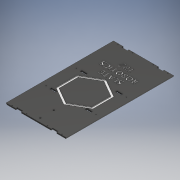
# Autodesk Inventor part: BA11
Saved by Autodesk Inventor 2017 (Build 210142000, 142)
## iProperties
Created: 2019-05-29
Part Number: BA11
Material: Wood (Cherry)
Document SubType Name: Modeling
Designer: Dell
Density: 0.63 g/cm^3
Appearance: Smooth - Black
Mass: 641.872 g
Surface Area: 3346.2 cm^2
Volume: 1018.84 cm^3
Author: Dell
Autodesk Inventor part; units mm, degrees
ref_plane "YZ Plane" through (0, 0, 0) normal (1, 0, 0) x (0, 1, 0)
ref_plane "XZ Plane" through (0, 0, 0) normal (0, 1, 0) x (-1, 0, 0)
ref_plane "XY Plane" through (0, 0, 0) normal (0, 0, 1) x (1, 0, 0)
sketch "Sketch1" plane through (0, 0, 0) normal (0, 0, 1) x (1, 0, 0)
  line L0 (0, 0) -> (303.5592, 0)
  line L1 (303.5592, 0) -> (303.5592, 539.75)
  line L2 (303.5592, 539.75) -> (0, 539.75)
  line L3 (0, 539.75) -> (0, 0)
  dimension "d0" = 539.75
  dimension "d1" = 303.5592
  constraints: 8 end point, 2 parallel, 1 horizontal, 1 perpendicular
  measures "d0" distance of L1.end L0.end
  measures "d1" distance of L1.end L2.end
extrude "Extrusion1" add sketch "Sketch1" along normal blind 6.35
sketch "Sketch2" plane through (0, 539.75, 0) normal (0, 1, 0) x (1, 0, 0)
  line L0 (0, -6.35) -> (303.5592, -6.35) projected
  line L1 (0, -6.35) -> (3.6662, 0)
  line L2 (0, 0) -> (303.5592, 0) projected
  line L3 (0, 0) -> (3.6662, 0)
  line L4 (0, 0) -> (0, -6.35)
  line L5 (303.5592, -6.35) -> (299.8931, 0)
  line L6 (303.5592, 0) -> (299.8931, 0)
  line L7 (303.5592, 0) -> (303.5592, -6.35) projected
  line L8 (303.5592, 0) -> (303.5592, -6.35)
  dimension "d4" = 30
  dimension "d5" = 30
  constraints: 12 end point, 2 collinear, 2 point on line, 1 perpendicular, 1 vertical
  measures "d4" angle of L4 L1
  measures "d5" angle of L5 L7
extrude "Extrusion2" cut sketch "Sketch2" against normal through all contours L4 L2 L1 | L5 L2 L7
sketch "Sketch3" plane through (0, 0, 6.35) normal (0, 0, 1) x (1, 0, 0)
  line L0 (50.1796, 532.13) -> (75.5796, 532.13)
  line L1 (75.5796, 532.13) -> (75.5796, 539.75)
  line L2 (75.5796, 539.75) -> (50.1796, 539.75)
  line L3 (50.1796, 539.75) -> (50.1796, 532.13)
  line L4 (303.5592, 539.75) -> (0, 539.75) projected
  line L5 (227.9796, 539.75) -> (253.3796, 539.75)
  line L6 (253.3796, 539.75) -> (253.3796, 532.13)
  line L7 (253.3796, 532.13) -> (227.9796, 532.13)
  line L8 (227.9796, 532.13) -> (227.9796, 539.75)
  line L9 (75.5796, 532.13) -> (227.9796, 532.13) construction
  line L10 (0, 0) -> (303.5592, 0) projected
  line L11 (50.1796, 0) -> (75.5796, 0)
  line L12 (75.5796, 0) -> (75.5796, 7.62)
  line L13 (75.5796, 7.62) -> (50.1796, 7.62)
  line L14 (50.1796, 7.62) -> (50.1796, 0)
  line L15 (253.3796, 0) -> (227.9796, 0)
  line L16 (227.9796, 0) -> (227.9796, 7.62)
  line L17 (227.9796, 7.62) -> (253.3796, 7.62)
  line L18 (253.3796, 7.62) -> (253.3796, 0)
  point P0 (151.7796, 532.13)
  point P1 (151.7796, 539.75)
  dimension "d8" = 7.62
  dimension "d9" = 25.4
  dimension "d10" = 25.4
  dimension "d11" = 152.4
  dimension "d14" = 7.62
  constraints: 34 end point, 8 parallel, 5 point on line, 5 vertical alignment, 4 horizontal, 4 perpendicular, 2 midpoint, 1 collinear, 1 horizontal alignment
  measures "d8" distance of L2.end L0.start
  measures "d9" distance of L0.start L0.end
  measures "d10" distance of L6.end L7.end
  measures "d11" distance of L0.end L7.end
  measures "d14" distance of L13.end L11.start
extrude "Extrusion3" cut sketch "Sketch3" against normal through all
sketch "Sketch4" plane through (0, 0, 6.35) normal (0, 0, 1) x (1, 0, 0)
  line L0 (50.1796, 330.2) -> (75.5796, 330.2)
  line L1 (75.5796, 330.2) -> (75.5796, 323.85)
  line L2 (75.5796, 323.85) -> (50.1796, 323.85)
  line L3 (50.1796, 323.85) -> (50.1796, 330.2)
  line L4 (227.9796, 330.2) -> (253.3796, 330.2)
  line L5 (253.3796, 330.2) -> (253.3796, 323.85)
  line L6 (253.3796, 323.85) -> (227.9796, 323.85)
  line L7 (227.9796, 323.85) -> (227.9796, 330.2)
  line L8 (75.5796, 532.13) -> (50.1796, 532.13) projected
  line L9 (253.3796, 532.13) -> (227.9796, 532.13) projected
  line L10 (227.9796, 539.75) -> (75.5796, 539.75) projected
  point P0 (0, 0)
  point P1 (62.8796, 330.2)
  point P2 (62.8796, 532.13)
  point P3 (240.6796, 330.2)
  point P4 (240.6796, 532.13)
  dimension "d15" = 25.4
  dimension "d16" = 6.35
  dimension "d17" = 25.4
  dimension "d18" = 6.35
  dimension "d19" = 209.55
  constraints: 16 end point, 4 midpoint, 4 parallel, 2 horizontal, 2 perpendicular, 2 vertical alignment, 1 horizontal alignment
  measures "d15" distance of L1.end L2.end
  measures "d16" distance of L0.end L1.end
  measures "d17" distance of L5.end L6.end
  measures "d18" distance of L4.end L5.end
  measures "d19" distance between parallel lines of L10 L0
extrude "Extrusion4" cut sketch "Sketch4" against normal through all
sketch "Sketch5" plane through (0, 0, 6.35) normal (0, 0, 1) x (1, 0, 0)
  line L0 (50.1796, 177.8) -> (75.5796, 177.8)
  line L1 (75.5796, 177.8) -> (75.5796, 171.45)
  line L2 (75.5796, 171.45) -> (50.1796, 171.45)
  line L3 (50.1796, 171.45) -> (50.1796, 177.8)
  line L4 (227.9796, 177.8) -> (253.3796, 177.8)
  line L5 (253.3796, 177.8) -> (253.3796, 171.45)
  line L6 (253.3796, 171.45) -> (227.9796, 171.45)
  line L7 (227.9796, 171.45) -> (227.9796, 177.8)
  line L8 (50.1796, 7.62) -> (75.5796, 7.62) projected
  line L9 (227.9796, 7.62) -> (253.3796, 7.62) projected
  line L10 (0, 0) -> (50.1796, 0) projected
  point P0 (62.8796, 171.45)
  point P1 (62.8796, 7.62)
  point P2 (240.6796, 7.62)
  point P3 (240.6796, 171.45)
  dimension "d22" = 25.4
  dimension "d23" = 6.35
  dimension "d24" = 25.4
  dimension "d25" = 6.35
  dimension "d27" = 177.8
  constraints: 16 end point, 4 midpoint, 4 parallel, 2 horizontal, 2 perpendicular, 2 vertical alignment, 1 horizontal alignment
  measures "d22" distance of L1.end L2.end
  measures "d23" distance of L0.end L1.end
  measures "d24" distance of L5.end L6.end
  measures "d25" distance of L4.end L5.end
  measures "d27" distance between parallel lines of L10 L0
extrude "Extrusion5" cut sketch "Sketch5" against normal through all
sketch "Sketch6" plane through (0, 0, 6.35) normal (0, 0, 1) x (1, 0, 0)
  line L0 (301.7796, 359.75) -> (1.7796, 359.75) construction
  line L1 (1.7796, 359.75) -> (1.7796, 469.75) construction
  line L2 (301.7796, 469.75) -> (301.7796, 359.75) construction
  line L3 (1.7796, 469.75) -> (301.7796, 469.75) construction
  line L4 (151.7796, 359.75) -> (151.7796, 414.75) construction
  line L5 (151.7796, 414.75) -> (1.7796, 414.75) construction
  line L6 (227.9796, 539.75) -> (75.5796, 539.75) projected
  line L7 (151.7796, 138.1902) -> (59.2796, 191.5951)
  line L8 (59.2796, 191.5951) -> (59.2796, 298.4049)
  line L9 (59.2796, 298.4049) -> (151.7796, 351.8098)
  line L10 (151.7796, 351.8098) -> (244.2796, 298.4049)
  line L11 (244.2796, 298.4049) -> (244.2796, 191.5951)
  line L12 (244.2796, 191.5951) -> (151.7796, 138.1902)
  line L13 (151.7796, 149.9681) -> (69.4796, 197.4841)
  line L14 (69.4796, 197.4841) -> (69.4796, 292.5159)
  line L15 (69.4796, 292.5159) -> (151.7796, 340.0319)
  line L16 (151.7796, 340.0319) -> (234.0796, 292.5159)
  line L17 (234.0796, 292.5159) -> (234.0796, 197.4841)
  line L18 (234.0796, 197.4841) -> (151.7796, 149.9681)
  line L19 (75.5796, 0) -> (227.9796, 0) projected
  line L20 (205.0313, 387.3542) -> (205.0313, 383.0696)
  spline S0 degree 2 poles (205.0313, 383.0696) (202.1048, 384.2937) (199.2165, 384.7719) (198.0114, 384.7719) knots 0 0 0 1 2 2 2
  spline S1 degree 2 poles (198.0114, 384.7719) (195.8309, 384.7719) (193.6694, 382.8209) (193.6694, 381.4437) knots 0 0 0 1 2 2 2
  spline S2 degree 2 poles (193.6694, 381.4437) (193.6694, 380.3917) (194.2624, 379.55) knots 0 0 0 1 1 1
  spline S3 degree 2 poles (194.2624, 379.55) (194.8745, 378.7276) (197.2272, 377.4077) knots 0 0 0 1 1 1
  line L21 (197.2272, 377.4077) -> (198.9104, 376.4705)
  spline S4 degree 2 poles (198.9104, 376.4705) (202.5256, 374.4621) (203.788, 372.7597) knots 0 0 0 1 1 1
  spline S5 degree 2 poles (203.788, 372.7597) (205.0887, 371.0573) (205.0887, 368.8194) knots 0 0 0 1 1 1
  spline S6 degree 2 poles (205.0887, 368.8194) (205.0887, 365.9885) (200.7658, 361.9716) (196.7299, 361.9716) knots 0 0 0 1 2 2 2
  spline S7 degree 2 poles (196.7299, 361.9716) (193.7077, 361.9716) (189.9204, 362.8324) knots 0 0 0 1 1 1
  line L22 (189.9204, 362.8324) -> (189.9204, 366.8301)
  spline S8 degree 2 poles (189.9204, 366.8301) (193.8033, 365.3955) (196.0795, 365.3955) knots 0 0 0 1 1 1
  spline S9 degree 2 poles (196.0795, 365.3955) (197.9732, 365.3955) (199.9433, 367.0405) (199.9433, 368.1882) knots 0 0 0 1 2 2 2
  spline S10 degree 2 poles (199.9433, 368.1882) (199.9433, 369.068) (199.3313, 369.814) knots 0 0 0 1 1 1
  spline S11 degree 2 poles (199.3313, 369.814) (198.7574, 370.5791) (196.4047, 371.8989) knots 0 0 0 1 1 1
  line L23 (196.4047, 371.8989) -> (194.6067, 372.8936)
  spline S12 degree 2 poles (194.6067, 372.8936) (190.456, 375.208) (189.3274, 376.9104) knots 0 0 0 1 1 1
  spline S13 degree 2 poles (189.3274, 376.9104) (188.1989, 378.6319) (188.1989, 380.7742) knots 0 0 0 1 1 1
  spline S14 degree 2 poles (188.1989, 380.7742) (188.1989, 383.8538) (192.8852, 388.1958) (197.9923, 388.1958) knots 0 0 0 1 2 2 2
  spline S15 degree 2 poles (197.9923, 388.1958) (201.0145, 388.1958) (205.0313, 387.3542) knots 0 0 0 1 1 1
  line L24 (183.876, 387.5837) -> (183.876, 362.5837)
  line L25 (183.876, 362.5837) -> (178.6733, 362.5837)
  line L26 (178.6733, 362.5837) -> (178.6733, 384.0451)
  line L27 (178.6733, 384.0451) -> (167.5218, 384.0451)
  line L28 (167.5218, 384.0451) -> (167.5218, 387.5837)
  line L29 (167.5218, 387.5837) -> (183.876, 387.5837)
  line L30 (166.508, 387.5837) -> (156.8102, 362.5837)
  line L31 (156.8102, 362.5837) -> (151.5883, 362.5837)
  line L32 (151.5883, 362.5837) -> (141.8523, 387.5837)
  line L33 (141.8523, 387.5837) -> (147.1889, 387.5837)
  line L34 (147.1889, 387.5837) -> (149.7903, 380.9081)
  line L35 (149.7903, 380.9081) -> (160.1193, 380.9081)
  line L36 (160.1193, 380.9081) -> (162.7207, 387.5837)
  line L37 (162.7207, 387.5837) -> (166.508, 387.5837)
  line L38 (158.8378, 377.5799) -> (151.091, 377.5799)
  line L39 (151.091, 377.5799) -> (154.9548, 367.6143)
  line L40 (154.9548, 367.6143) -> (158.8378, 377.5799)
  line L41 (132.0971, 387.5837) -> (132.0971, 366.0267)
  line L42 (132.0971, 366.0267) -> (141.0489, 366.0267)
  line L43 (141.0489, 366.0267) -> (141.0489, 362.5837)
  line L44 (141.0489, 362.5837) -> (117.9426, 362.5837)
  line L45 (117.9426, 362.5837) -> (117.9426, 366.0267)
  line L46 (117.9426, 366.0267) -> (126.8944, 366.0267)
  line L47 (126.8944, 366.0267) -> (126.8944, 387.5837)
  line L48 (126.8944, 387.5837) -> (132.0971, 387.5837)
  line L49 (114.4613, 387.5837) -> (114.4613, 362.5837)
  line L50 (114.4613, 362.5837) -> (98.4514, 362.5837)
  line L51 (98.4514, 362.5837) -> (98.4514, 366.0267)
  line L52 (98.4514, 366.0267) -> (109.2586, 366.0267)
  line L53 (109.2586, 366.0267) -> (109.2586, 372.9892)
  line L54 (109.2586, 372.9892) -> (100.3259, 372.9892)
  line L55 (100.3259, 372.9892) -> (100.3259, 376.4322)
  line L56 (100.3259, 376.4322) -> (109.2586, 376.4322)
  line L57 (109.2586, 376.4322) -> (109.2586, 384.0451)
  line L58 (109.2586, 384.0451) -> (97.648, 384.0451)
  line L59 (97.648, 384.0451) -> (97.648, 387.5837)
  line L60 (97.648, 387.5837) -> (114.4613, 387.5837)
  line L61 (239.7961, 427.5402) -> (239.7961, 402.5402)
  line L62 (239.7961, 402.5402) -> (230.4426, 402.5402)
  spline S16 degree 2 poles (230.4426, 402.5402) (227.5734, 402.5402) (224.5703, 403.9748) (222.8297, 406.9014) (222.8297, 408.7376) knots 0 0 0 1 2 3 3 3
  spline S17 degree 2 poles (222.8297, 408.7376) (222.8297, 410.9373) (225.3546, 414.8394) (227.669, 415.8723) knots 0 0 0 1 2 2 2
  line L63 (227.669, 415.8723) -> (219.5015, 427.5402)
  line L64 (219.5015, 427.5402) -> (225.8328, 427.5402)
  line L65 (225.8328, 427.5402) -> (232.0493, 417.326)
  line L66 (232.0493, 417.326) -> (234.8993, 417.326)
  line L67 (234.8993, 417.326) -> (234.8993, 427.5402)
  line L68 (234.8993, 427.5402) -> (239.7961, 427.5402)
  line L69 (234.8993, 413.9021) -> (233.7134, 413.9021)
  spline S18 degree 2 poles (233.7134, 413.9021) (230.5, 413.9021) (228.0325, 411.0903) (228.0325, 409.3115) knots 0 0 0 1 2 2 2
  spline S19 degree 2 poles (228.0325, 409.3115) (228.0325, 407.7812) (230.0218, 405.9641) (233.0822, 405.9641) knots 0 0 0 1 2 2 2
  line L70 (233.0822, 405.9641) -> (234.8993, 405.9641)
  line L71 (234.8993, 405.9641) -> (234.8993, 413.9021)
  spline S20 degree 2 poles (204.8114, 428.1523) (208.7134, 428.1523) (214.49, 424.9197) (217.4931, 418.8753) (217.4931, 415.0307) knots 0 0 0 1 2 3 3 3
  spline S21 degree 2 poles (217.4931, 415.0307) (217.4931, 411.2242) (214.49, 405.1416) (208.6752, 401.9281) (204.8114, 401.9281) knots 0 0 0 1 2 3 3 3
  spline S22 degree 2 poles (204.8114, 401.9281) (200.9667, 401.9281) (195.1518, 405.1416) (192.1488, 411.2242) (192.1488, 415.0307) knots 0 0 0 1 2 3 3 3
  spline S23 degree 2 poles (192.1488, 415.0307) (192.1488, 418.8753) (195.1518, 424.9197) (200.9093, 428.1523) (204.8114, 428.1523) knots 0 0 0 1 2 3 3 3
  spline S24 degree 2 poles (204.8114, 424.7284) (201.1962, 424.7284) (197.6767, 418.8371) (197.6767, 415.0307) knots 0 0 0 1 2 2 2
  spline S25 degree 2 poles (197.6767, 415.0307) (197.6767, 411.2051) (201.2153, 405.352) (204.8114, 405.352) knots 0 0 0 1 2 2 2
  spline S26 degree 2 poles (204.8114, 405.352) (208.4265, 405.352) (211.9651, 411.2051) (211.9651, 415.0307) knots 0 0 0 1 2 2 2
  spline S27 degree 2 poles (211.9651, 415.0307) (211.9651, 418.8371) (208.4456, 424.7284) (204.8114, 424.7284) knots 0 0 0 1 2 2 2
  line L72 (187.4816, 427.5402) -> (187.4816, 402.5402)
  line L73 (187.4816, 402.5402) -> (179.0462, 402.5402)
  spline S28 degree 2 poles (179.0462, 402.5402) (175.9858, 402.5402) (173.0593, 403.9174) (171.3951, 406.5953) (171.3951, 408.1064) knots 0 0 0 1 2 3 3 3
  spline S29 degree 2 poles (171.3951, 408.1064) (171.3951, 409.9809) (173.9965, 413.4239) (177.363, 414.476) knots 0 0 0 1 2 2 2
  spline S30 degree 2 poles (177.363, 414.476) (174.6851, 415.1454) (171.8542, 417.0965) (170.3814, 419.8126) (170.3814, 421.362) knots 0 0 0 1 2 3 3 3
  spline S31 degree 2 poles (170.3814, 421.362) (170.3814, 423.0452) (172.1029, 425.9717) (175.1251, 427.5402) (178.262, 427.5402) knots 0 0 0 1 2 3 3 3
  line L74 (178.262, 427.5402) -> (187.4816, 427.5402)
  line L75 (182.4892, 424.0016) -> (181.4946, 424.0016)
  spline S32 degree 2 poles (181.4946, 424.0016) (178.7785, 424.0016) (176.8083, 423.2939) (175.8137, 421.7063) (175.8137, 420.7307) knots 0 0 0 1 2 3 3 3
  spline S33 degree 2 poles (175.8137, 420.7307) (175.8137, 418.8753) (179.0845, 416.2931) (181.5902, 416.2931) knots 0 0 0 1 2 2 2
  line L76 (181.5902, 416.2931) -> (182.4892, 416.2931)
  line L77 (182.4892, 416.2931) -> (182.4892, 424.0016)
  line L78 (182.4892, 412.9457) -> (181.3798, 412.9457)
  spline S34 degree 2 poles (181.3798, 412.9457) (179.008, 412.9457) (176.6744, 410.593) (176.6744, 408.9098) knots 0 0 0 1 2 2 2
  spline S35 degree 2 poles (176.6744, 408.9098) (176.6744, 408.0108) (177.363, 406.6909) (179.1036, 405.9641) (181.552, 405.9641) knots 0 0 0 1 2 3 3 3
  line L79 (181.552, 405.9641) -> (182.4892, 405.9641)
  line L80 (182.4892, 405.9641) -> (182.4892, 412.9457)
  spline S36 degree 2 poles (154.5627, 428.1523) (158.4648, 428.1523) (164.2414, 424.9197) (167.2444, 418.8753) (167.2444, 415.0307) knots 0 0 0 1 2 3 3 3
  spline S37 degree 2 poles (167.2444, 415.0307) (167.2444, 411.2242) (164.2414, 405.1416) (158.4265, 401.9281) (154.5627, 401.9281) knots 0 0 0 1 2 3 3 3
  spline S38 degree 2 poles (154.5627, 401.9281) (150.718, 401.9281) (144.9032, 405.1416) (141.9001, 411.2242) (141.9001, 415.0307) knots 0 0 0 1 2 3 3 3
  spline S39 degree 2 poles (141.9001, 415.0307) (141.9001, 418.8753) (144.9032, 424.9197) (150.6606, 428.1523) (154.5627, 428.1523) knots 0 0 0 1 2 3 3 3
  spline S40 degree 2 poles (154.5627, 424.7284) (150.9475, 424.7284) (147.428, 418.8371) (147.428, 415.0307) knots 0 0 0 1 2 2 2
  spline S41 degree 2 poles (147.428, 415.0307) (147.428, 411.2051) (150.9667, 405.352) (154.5627, 405.352) knots 0 0 0 1 2 2 2
  spline S42 degree 2 poles (154.5627, 405.352) (158.1778, 405.352) (161.7165, 411.2051) (161.7165, 415.0307) knots 0 0 0 1 2 2 2
  spline S43 degree 2 poles (161.7165, 415.0307) (161.7165, 418.8371) (158.197, 424.7284) (154.5627, 424.7284) knots 0 0 0 1 2 2 2
  line L81 (131.0164, 427.5402) -> (131.0164, 405.9832)
  line L82 (131.0164, 405.9832) -> (139.9682, 405.9832)
  line L83 (139.9682, 405.9832) -> (139.9682, 402.5402)
  line L84 (139.9682, 402.5402) -> (116.8619, 402.5402)
  line L85 (116.8619, 402.5402) -> (116.8619, 405.9832)
  line L86 (116.8619, 405.9832) -> (125.8137, 405.9832)
  line L87 (125.8137, 405.9832) -> (125.8137, 427.5402)
  line L88 (125.8137, 427.5402) -> (131.0164, 427.5402)
  line L89 (113.3806, 427.5402) -> (113.3806, 402.5402)
  line L90 (113.3806, 402.5402) -> (108.1778, 402.5402)
  line L91 (108.1778, 402.5402) -> (108.1778, 427.5402)
  line L92 (108.1778, 427.5402) -> (113.3806, 427.5402)
  spline S44 degree 2 poles (81.8006, 426.5456) (83.4456, 427.2724) (85.8749, 427.808) (88.9544, 428.1523) (90.4655, 428.1523) knots 0 0 0 1 2 3 3 3
  spline S45 degree 2 poles (90.4655, 428.1523) (97.0264, 428.1523) (103.4724, 420.769) (103.4724, 415.0307) knots 0 0 0 1 2 2 2
  spline S46 degree 2 poles (103.4724, 415.0307) (103.4724, 409.2923) (97.0455, 401.9281) (90.1404, 401.9281) knots 0 0 0 1 2 2 2
  spline S47 degree 2 poles (90.1404, 401.9281) (86.0661, 401.9281) (82.0302, 402.8845) knots 0 0 0 1 1 1
  line L93 (82.0302, 402.8845) -> (82.0302, 406.9587)
  spline S48 degree 2 poles (82.0302, 406.9587) (83.9812, 406.2893) (86.4487, 405.658) (88.6484, 405.352) (89.7578, 405.352) knots 0 0 0 1 2 3 3 3
  spline S49 degree 2 poles (89.7578, 405.352) (94.0616, 405.352) (97.9445, 410.8799) (97.9445, 414.9733) knots 0 0 0 1 2 2 2
  spline S50 degree 2 poles (97.9445, 414.9733) (97.9445, 419.2579) (93.5451, 424.5563) (89.184, 424.5563) knots 0 0 0 1 2 2 2
  spline S51 degree 2 poles (89.184, 424.5563) (85.5497, 424.5563) (81.8006, 422.72) knots 0 0 0 1 1 1
  line L94 (81.8006, 422.72) -> (81.8006, 426.5456)
  line L95 (78.6828, 427.3107) -> (78.6828, 423.0261)
  spline S52 degree 2 poles (78.6828, 423.0261) (75.7563, 424.2502) (72.868, 424.7284) (71.6629, 424.7284) knots 0 0 0 1 2 2 2
  spline S53 degree 2 poles (71.6629, 424.7284) (69.4824, 424.7284) (67.3209, 422.7774) (67.3209, 421.4002) knots 0 0 0 1 2 2 2
  spline S54 degree 2 poles (67.3209, 421.4002) (67.3209, 420.3482) (67.9139, 419.5066) knots 0 0 0 1 1 1
  spline S55 degree 2 poles (67.9139, 419.5066) (68.526, 418.6841) (70.8787, 417.3642) knots 0 0 0 1 1 1
  line L96 (70.8787, 417.3642) -> (72.5619, 416.427)
  spline S56 degree 2 poles (72.5619, 416.427) (76.1771, 414.4186) (77.4395, 412.7162) knots 0 0 0 1 1 1
  spline S57 degree 2 poles (77.4395, 412.7162) (78.7402, 411.0138) (78.7402, 408.7759) knots 0 0 0 1 1 1
  spline S58 degree 2 poles (78.7402, 408.7759) (78.7402, 405.945) (74.4173, 401.9281) (70.3814, 401.9281) knots 0 0 0 1 2 2 2
  spline S59 degree 2 poles (70.3814, 401.9281) (67.3592, 401.9281) (63.5719, 402.7889) knots 0 0 0 1 1 1
  line L97 (63.5719, 402.7889) -> (63.5719, 406.7866)
  spline S60 degree 2 poles (63.5719, 406.7866) (67.4548, 405.352) (69.731, 405.352) knots 0 0 0 1 1 1
  spline S61 degree 2 poles (69.731, 405.352) (71.6247, 405.352) (73.5948, 406.997) (73.5948, 408.1447) knots 0 0 0 1 2 2 2
  spline S62 degree 2 poles (73.5948, 408.1447) (73.5948, 409.0245) (72.9827, 409.7705) knots 0 0 0 1 1 1
  spline S63 degree 2 poles (72.9827, 409.7705) (72.4089, 410.5356) (70.0562, 411.8554) knots 0 0 0 1 1 1
  line L98 (70.0562, 411.8554) -> (68.2582, 412.8501)
  spline S64 degree 2 poles (68.2582, 412.8501) (64.1075, 415.1646) (62.9789, 416.8669) knots 0 0 0 1 1 1
  spline S65 degree 2 poles (62.9789, 416.8669) (61.8504, 418.5884) (61.8504, 420.7307) knots 0 0 0 1 1 1
  spline S66 degree 2 poles (61.8504, 420.7307) (61.8504, 423.8103) (66.5367, 428.1523) (71.6438, 428.1523) knots 0 0 0 1 2 2 2
  spline S67 degree 2 poles (71.6438, 428.1523) (74.666, 428.1523) (78.6828, 427.3107) knots 0 0 0 1 1 1
  line L99 (175.4335, 467.5284) -> (170.9719, 445.1822)
  line L100 (170.9719, 445.1822) -> (179.8565, 445.1822)
  line L101 (179.8565, 445.1822) -> (179.3373, 442.5284)
  line L102 (179.3373, 442.5284) -> (158.0488, 442.5284)
  line L103 (158.0488, 442.5284) -> (158.5873, 445.1822)
  line L104 (158.5873, 445.1822) -> (167.4527, 445.1822)
  line L105 (167.4527, 445.1822) -> (171.895, 467.5284)
  line L106 (171.895, 467.5284) -> (175.4335, 467.5284)
  line L107 (159.645, 467.5284) -> (154.6642, 442.5284)
  line L108 (154.6642, 442.5284) -> (147.1258, 442.5284)
  spline S68 degree 2 poles (147.1258, 442.5284) (145.145, 442.5284) (142.4335, 443.2015) (140.645, 445.6245) (140.645, 447.3745) knots 0 0 0 1 2 3 3 3
  spline S69 degree 2 poles (140.645, 447.3745) (140.645, 449.913) (144.2604, 454.413) (147.3373, 455.5861) knots 0 0 0 1 2 2 2
  line L109 (147.3373, 455.5861) -> (141.395, 467.5284)
  line L110 (141.395, 467.5284) -> (145.3181, 467.5284)
  line L111 (145.3181, 467.5284) -> (150.5681, 456.4707)
  line L112 (150.5681, 456.4707) -> (153.9142, 456.4707)
  line L113 (153.9142, 456.4707) -> (156.1065, 467.5284)
  line L114 (156.1065, 467.5284) -> (159.645, 467.5284)
  line L115 (153.395, 453.8553) -> (151.4335, 453.8553)
  spline S70 degree 2 poles (151.4335, 453.8553) (149.3373, 453.8553) (146.2412, 452.2784) (144.4142, 449.2784) (144.4142, 447.7784) knots 0 0 0 1 2 3 3 3
  spline S71 degree 2 poles (144.4142, 447.7784) (144.4142, 446.4899) (146.3758, 445.1822) (149.4142, 445.1822) knots 0 0 0 1 2 2 2
  line L116 (149.4142, 445.1822) -> (151.6642, 445.1822)
  line L117 (151.6642, 445.1822) -> (153.395, 453.8553)
  line L118 (137.7027, 467.5284) -> (137.1642, 464.8361)
  spline S72 degree 2 poles (137.1642, 464.8361) (136.0296, 462.7591) (132.8181, 459.4515) (130.4719, 457.6438) knots 0 0 0 1 2 2 2
  line L119 (130.4719, 457.6438) -> (128.3758, 456.0476)
  spline S73 degree 2 poles (128.3758, 456.0476) (125.395, 453.7591) (123.7988, 451.8168) knots 0 0 0 1 1 1
  spline S74 degree 2 poles (123.7988, 451.8168) (122.9912, 450.8361) (122.1835, 448.8938) (122.1835, 447.9322) knots 0 0 0 1 2 2 2
  spline S75 degree 2 poles (122.1835, 447.9322) (122.1835, 446.3553) (124.3565, 444.413) (126.4912, 444.413) knots 0 0 0 1 2 2 2
  spline S76 degree 2 poles (126.4912, 444.413) (129.4912, 444.413) (133.0873, 446.4515) knots 0 0 0 1 1 1
  line L120 (133.0873, 446.4515) -> (132.4912, 443.4707)
  spline S77 degree 2 poles (132.4912, 443.4707) (131.9142, 443.2591) (131.645, 443.1245) knots 0 0 0 1 1 1
  spline S78 degree 2 poles (131.645, 443.1245) (128.3565, 441.913) (125.645, 441.913) knots 0 0 0 1 1 1
  spline S79 degree 2 poles (125.645, 441.913) (122.4527, 441.913) (118.645, 444.7015) (118.645, 447.5284) knots 0 0 0 1 2 2 2
  spline S80 degree 2 poles (118.645, 447.5284) (118.645, 449.0284) (119.1835, 450.3553) knots 0 0 0 1 1 1
  spline S81 degree 2 poles (119.1835, 450.3553) (119.9912, 452.3938) (122.9335, 455.2399) (125.645, 457.2207) knots 0 0 0 1 2 2 2
  line L121 (125.645, 457.2207) -> (127.7412, 458.7399)
  spline S82 degree 2 poles (127.7412, 458.7399) (129.6258, 460.1245) (131.0296, 461.4322) (131.6835, 462.2207) knots 0 0 0 1 2 2 2
  spline S83 degree 2 poles (131.6835, 462.2207) (132.0681, 462.7207) (132.7796, 463.6822) (133.1835, 464.6245) knots 0 0 0 1 2 2 2
  line L122 (133.1835, 464.6245) -> (122.2219, 464.6245)
  line L123 (122.2219, 464.6245) -> (122.8181, 467.5284)
  line L124 (122.8181, 467.5284) -> (137.7027, 467.5284)
  point P0 (0, 0)
  point P1 (151.7796, 469.75)
  point P2 (151.7796, 539.75)
  point P3 (151.7796, 245)
  dimension "d32" = 300
  dimension "d34" = 185
  dimension "d35" = 10.2
  dimension "d38" = 245
  dimension "d39" = 125
  dimension "d40" = 110
  constraints: 28 end point, 4 midpoint, 2 horizontal, 2 vertical, 2 vertical alignment, 20 other
  measures "d32" distance of L2.end L0.end
  measures "d34" distance between parallel lines of L11 L8
  measures "d35" distance between parallel lines of L12 L18
  measures "d38" distance from line of point (151.78, 245) L19
  measures "d39" distance from line of L6 L4.end
  measures "d40" distance of L2.start L2.end
extrude "Extrusion6" cut sketch "Sketch6" against normal blind 3.175
sketch "Sketch7" plane through (0, 0, 6.35) normal (0, 0, 1) x (1, 0, 0)
  line L0 (26.2013, 535.94) -> (99.558, 535.94) construction
  line L1 (75.5796, 532.13) -> (50.1796, 532.13) construction
  line L2 (50.1796, 532.13) -> (50.1796, 539.75) construction
  line L3 (204.0013, 535.94) -> (277.358, 535.94) construction
  line L4 (253.3796, 532.13) -> (227.9796, 532.13) construction
  circle A0 centre (26.2013, 535.94) radius 2.25
  circle A1 centre (99.558, 535.94) radius 2.25
  circle A2 centre (204.0013, 535.94) radius 2.25
  circle A3 centre (277.358, 535.94) radius 2.25
  circle A4 centre (26.2013, 327.025) radius 2.25
  circle A5 centre (99.558, 327.025) radius 2.25
  circle A6 centre (204.0013, 327.025) radius 2.25
  circle A7 centre (277.358, 327.025) radius 2.25
  circle A8 centre (277.358, 174.625) radius 2.25
  circle A9 centre (26.2013, 174.625) radius 2.25
  circle A10 centre (151.7796, 174.625) radius 2.25
  circle A11 centre (26.2013, 3.81) radius 2.25
  circle A12 centre (99.558, 3.81) radius 2.25
  circle A13 centre (204.0013, 3.81) radius 2.25
  circle A14 centre (277.358, 3.81) radius 2.25
  line L5 (227.9796, 539.75) -> (75.5796, 539.75) projected
  line L6 (50.1796, 323.85) -> (50.1796, 330.2) projected
  line L7 (50.1796, 171.45) -> (50.1796, 177.8) projected
  line L8 (50.1796, 0) -> (50.1796, 7.62) projected
  point P0 (0, 0)
  point P1 (62.8796, 535.94)
  point P2 (62.8796, 532.13)
  point P3 (50.1796, 535.94)
  point P4 (240.6796, 535.94)
  point P5 (240.6796, 532.13)
  point P6 (151.7796, 539.75)
  point P7 (50.1796, 327.025)
  point P8 (50.1796, 174.625)
  point P9 (50.1796, 3.81)
  dimension "d41" = 73.3567
  dimension "d42" = 73.3567
  dimension "d43" = 4.5
  dimension "d44" = 4.5
  dimension "d45" = 4.5
  dimension "d46" = 4.5
  dimension "d47" = 4.5
  dimension "d48" = 4.5
  dimension "d49" = 4.5
  dimension "d50" = 4.5
  dimension "d51" = 4.5
  dimension "d52" = 4.5
  dimension "d53" = 4.5
  dimension "d54" = 4.5
  dimension "d55" = 4.5
  dimension "d56" = 4.5
  dimension "d57" = 4.5
  constraints: 15 centre point, 13 horizontal alignment, 13 vertical alignment, 9 midpoint, 4 coincident, 4 end point, 2 horizontal
  measures "d41" distance of L0.start L0.end
  measures "d42" distance of L3.start L3.end
  measures "d43" diameter of A0
  measures "d44" diameter of A1
  measures "d45" diameter of A2
  measures "d46" diameter of A3
  measures "d47" diameter of A4
  measures "d48" diameter of A5
  measures "d49" diameter of A6
  measures "d50" diameter of A7
  measures "d51" diameter of A8
  measures "d52" diameter of A9
  measures "d53" diameter of A10
  measures "d54" diameter of A11
  measures "d55" diameter of A12
  measures "d56" diameter of A13
  measures "d57" diameter of A14
extrude "Extrusion7" cut sketch "Sketch7" against normal through all contours A0 | A1 | A2 | A3 | A4 | A7 | A8 | A9 | A11 | A12 | A13 | A14
sketch "Sketch8" plane through (0, 0, 6.35) normal (0, 0, 1) x (1, 0, 0)
  circle A0 centre (151.7796, 20) radius 4
  circle A1 centre (151.7796, 87.71) radius 4
  line L0 (75.5796, 0) -> (227.9796, 0) projected
  point P0 (0, 0)
  point P1 (151.7796, 0)
  point P2 (151.7796, 0)
  dimension "d60" = 8
  dimension "d61" = 8
  dimension "d63" = 20
  dimension "d64" = 67.71
  constraints: 2 centre point, 2 midpoint, 2 vertical alignment
  measures "d60" diameter of A0
  measures "d61" diameter of A1
  measures "d63" distance from line of L0 A0.centre
  measures "d64" distance of A1.centre A0.centre
extrude "Extrusion8" cut sketch "Sketch8" against normal through all
sketch "Sketch9" plane through (0, 0, 6.35) normal (0, 0, 1) x (1, 0, 0)
  line L0 (50.1796, 539.75) -> (3.6662, 539.75) projected
  line L1 (48.9096, 539.75) -> (76.8496, 539.75)
  line L2 (76.8496, 539.75) -> (76.8496, 532.13)
  line L3 (76.8496, 532.13) -> (48.9096, 532.13)
  line L4 (48.9096, 532.13) -> (48.9096, 539.75)
  line L5 (227.9796, 539.75) -> (75.5796, 539.75) projected
  line L6 (226.7096, 539.75) -> (254.6496, 539.75)
  line L7 (254.6496, 539.75) -> (254.6496, 532.13)
  line L8 (254.6496, 532.13) -> (226.7096, 532.13)
  line L9 (226.7096, 532.13) -> (226.7096, 539.75)
  line L10 (48.9096, 331.47) -> (76.8496, 331.47)
  line L11 (76.8496, 331.47) -> (76.8496, 322.58)
  line L12 (76.8496, 322.58) -> (48.9096, 322.58)
  line L13 (48.9096, 322.58) -> (48.9096, 331.47)
  line L14 (48.9096, 179.07) -> (76.8496, 179.07)
  line L15 (76.8496, 179.07) -> (76.8496, 170.18)
  line L16 (76.8496, 170.18) -> (48.9096, 170.18)
  line L17 (48.9096, 170.18) -> (48.9096, 179.07)
  line L18 (254.6496, 170.18) -> (226.7096, 170.18)
  line L19 (226.7096, 170.18) -> (226.7096, 179.07)
  line L20 (226.7096, 179.07) -> (254.6496, 179.07)
  line L21 (254.6496, 179.07) -> (254.6496, 170.18)
  line L22 (254.6496, 322.58) -> (226.7096, 322.58)
  line L23 (226.7096, 322.58) -> (226.7096, 331.47)
  line L24 (226.7096, 331.47) -> (254.6496, 331.47)
  line L25 (254.6496, 331.47) -> (254.6496, 322.58)
  line L26 (3.6662, 0) -> (50.1796, 0) projected
  line L27 (48.9096, 0) -> (76.8496, 0)
  line L28 (76.8496, 0) -> (76.8496, 7.62)
  line L29 (76.8496, 7.62) -> (48.9096, 7.62)
  line L30 (48.9096, 7.62) -> (48.9096, 0)
  line L31 (75.5796, 0) -> (227.9796, 0) projected
  line L32 (226.7096, 0) -> (254.6496, 0)
  line L33 (254.6496, 0) -> (254.6496, 7.62)
  line L34 (254.6496, 7.62) -> (226.7096, 7.62)
  line L35 (226.7096, 7.62) -> (226.7096, 0)
  line L36 (50.1796, 7.62) -> (75.5796, 7.62) projected
  line L37 (227.9796, 7.62) -> (253.3796, 7.62) projected
  line L38 (253.3796, 532.13) -> (227.9796, 532.13) projected
  line L39 (75.5796, 532.13) -> (50.1796, 532.13) projected
  line L40 (50.1796, 532.13) -> (50.1796, 539.75) projected
  line L41 (227.9796, 532.13) -> (227.9796, 539.75) projected
  line L42 (227.9796, 0) -> (227.9796, 7.62) projected
  line L43 (50.1796, 0) -> (50.1796, 7.62) projected
  line L44 (50.1796, 177.8) -> (75.5796, 177.8) projected
  line L45 (227.9796, 177.8) -> (253.3796, 177.8) projected
  line L46 (50.1796, 330.2) -> (75.5796, 330.2) projected
  line L47 (227.9796, 323.85) -> (227.9796, 330.2) projected
  line L48 (75.5796, 330.2) -> (75.5796, 323.85) projected
  line L49 (227.9796, 171.45) -> (227.9796, 177.8) projected
  line L50 (75.5796, 177.8) -> (75.5796, 171.45) projected
  line L51 (227.9796, 330.2) -> (253.3796, 330.2) projected
  point P0 (0, 0)
  point P1 (62.8796, 7.62)
  point P2 (62.8796, 7.62)
  point P3 (240.6796, 7.62)
  point P4 (240.6796, 532.13)
  point P5 (62.8796, 532.13)
  point P6 (75.5796, 327.025)
  point P7 (76.8496, 327.025)
  point P8 (227.9796, 174.625)
  point P9 (226.7096, 174.625)
  point P10 (75.5796, 174.625)
  point P11 (76.8496, 174.625)
  point P12 (62.8796, 330.2)
  point P13 (62.8796, 331.47)
  point P14 (240.6796, 330.2)
  point P15 (240.6796, 331.47)
  point P16 (62.8796, 177.8)
  point P17 (62.8796, 179.07)
  point P18 (62.8796, 177.8)
  dimension "d68" = 1.27
  dimension "d69" = 1.27
  dimension "d70" = 1.27
  dimension "d71" = 1.27
  dimension "d72" = 1.27
  dimension "d73" = 1.27
  dimension "d74" = 1.27
  dimension "d75" = 1.27
  constraints: 64 end point, 23 midpoint, 16 parallel, 11 point on line, 8 horizontal, 8 perpendicular, 3 horizontal alignment, 3 vertical alignment
  measures "d68" distance between parallel lines of L4 L40
  measures "d69" distance between parallel lines of L41 L9
  measures "d70" distance between parallel lines of L42 L35
  measures "d71" distance between parallel lines of L30 L43
  measures "d72" distance between parallel lines of L14 L44
  measures "d73" distance between parallel lines of L20 L45
  measures "d74" distance between parallel lines of L10 L46
  measures "d75" distance between parallel lines of L23 L47
extrude "Extrusion9" cut sketch "Sketch9" against normal through all
sketch "Sketch10" plane through (0, 0, 6.35) normal (0, 0, 1) x (1, 0, 0)
  line L0 (76.8496, 7.62) -> (76.8496, 0) construction
  line L1 (76.8496, 0) -> (226.7096, 0) construction
  line L2 (226.7096, 0) -> (226.7096, 7.62) construction
  line L3 (226.7096, 7.62) -> (254.6496, 7.62) construction
  line L4 (254.6496, 7.62) -> (254.6496, 0) construction
  line L5 (254.6496, 0) -> (303.5592, 0) construction
  line L6 (303.5592, 0) -> (303.5592, 539.75) construction
  line L7 (303.5592, 539.75) -> (254.6496, 539.75) construction
  line L8 (254.6496, 539.75) -> (254.6496, 532.13) construction
  line L9 (254.6496, 532.13) -> (226.7096, 532.13) construction
  line L10 (226.7096, 532.13) -> (226.7096, 539.75) construction
  line L11 (226.7096, 539.75) -> (76.8496, 539.75) construction
  line L12 (76.8496, 539.75) -> (76.8496, 532.13) construction
  line L13 (76.8496, 532.13) -> (48.9096, 532.13) construction
  line L14 (48.9096, 532.13) -> (48.9096, 539.75) construction
  line L15 (48.9096, 539.75) -> (0, 539.75) construction
  line L16 (0, 539.75) -> (0, 0) construction
  line L17 (0, 0) -> (48.9096, 0) construction
  line L18 (48.9096, 0) -> (48.9096, 7.62) construction
  line L19 (48.9096, 7.62) -> (76.8496, 7.62) construction
  line L20 (254.6496, 179.07) -> (254.6496, 170.18) construction
  line L21 (254.6496, 170.18) -> (226.7096, 170.18) construction
  line L22 (226.7096, 170.18) -> (226.7096, 179.07) construction
  line L23 (226.7096, 179.07) -> (254.6496, 179.07) construction
  line L24 (48.9096, 322.58) -> (48.9096, 331.47) construction
  line L25 (48.9096, 331.47) -> (76.8496, 331.47) construction
  line L26 (76.8496, 331.47) -> (76.8496, 322.58) construction
  line L27 (76.8496, 322.58) -> (48.9096, 322.58) construction
  line L28 (48.9096, 170.18) -> (48.9096, 179.07) construction
  line L29 (48.9096, 179.07) -> (76.8496, 179.07) construction
  line L30 (76.8496, 179.07) -> (76.8496, 170.18) construction
  line L31 (76.8496, 170.18) -> (48.9096, 170.18) construction
  line L32 (254.6496, 331.47) -> (254.6496, 322.58) construction
  line L33 (254.6496, 322.58) -> (226.7096, 322.58) construction
  line L34 (226.7096, 322.58) -> (226.7096, 331.47) construction
  line L35 (226.7096, 331.47) -> (254.6496, 331.47) construction
  circle A0 centre (151.7796, 20) radius 4 construction
  circle A1 centre (151.7796, 87.71) radius 4 construction
  circle A2 centre (204.0013, 3.81) radius 2.25 construction
  circle A3 centre (26.2013, 3.81) radius 2.25 construction
  circle A4 centre (277.358, 174.625) radius 2.25 construction
  circle A5 centre (26.2013, 327.025) radius 2.25 construction
  circle A6 centre (204.0013, 535.94) radius 2.25 construction
  circle A7 centre (26.2013, 535.94) radius 2.25 construction
  circle A8 centre (99.558, 535.94) radius 2.25 construction
  circle A9 centre (277.358, 535.94) radius 2.25 construction
  circle A10 centre (277.358, 327.025) radius 2.25 construction
  circle A11 centre (26.2013, 174.625) radius 2.25 construction
  circle A12 centre (99.558, 3.81) radius 2.25 construction
  circle A13 centre (277.358, 3.81) radius 2.25 construction
  line L36 (171.895, 467.5284) -> (175.4335, 467.5284) construction
  line L37 (175.4335, 467.5284) -> (170.9719, 445.1822) construction
  line L38 (170.9719, 445.1822) -> (179.8565, 445.1822) construction
  line L39 (179.8565, 445.1822) -> (179.3373, 442.5284) construction
  line L40 (179.3373, 442.5284) -> (158.0488, 442.5284) construction
  line L41 (158.0488, 442.5284) -> (158.5873, 445.1822) construction
  line L42 (158.5873, 445.1822) -> (167.4527, 445.1822) construction
  line L43 (167.4527, 445.1822) -> (171.895, 467.5284) construction
  line L44 (81.8006, 422.72) -> (81.8006, 426.5456) construction
  line L45 (82.0302, 402.8845) -> (82.0302, 406.9587) construction
  line L46 (125.8137, 427.5402) -> (131.0164, 427.5402) construction
  line L47 (131.0164, 427.5402) -> (131.0164, 405.9832) construction
  line L48 (131.0164, 405.9832) -> (139.9682, 405.9832) construction
  line L49 (139.9682, 405.9832) -> (139.9682, 402.5402) construction
  line L50 (139.9682, 402.5402) -> (116.8619, 402.5402) construction
  line L51 (116.8619, 402.5402) -> (116.8619, 405.9832) construction
  line L52 (116.8619, 405.9832) -> (125.8137, 405.9832) construction
  line L53 (125.8137, 405.9832) -> (125.8137, 427.5402) construction
  line L54 (97.648, 387.5837) -> (114.4613, 387.5837) construction
  line L55 (114.4613, 387.5837) -> (114.4613, 362.5837) construction
  line L56 (114.4613, 362.5837) -> (98.4514, 362.5837) construction
  line L57 (98.4514, 362.5837) -> (98.4514, 366.0267) construction
  line L58 (98.4514, 366.0267) -> (109.2586, 366.0267) construction
  line L59 (109.2586, 366.0267) -> (109.2586, 372.9892) construction
  line L60 (109.2586, 372.9892) -> (100.3259, 372.9892) construction
  line L61 (100.3259, 372.9892) -> (100.3259, 376.4322) construction
  line L62 (100.3259, 376.4322) -> (109.2586, 376.4322) construction
  line L63 (109.2586, 376.4322) -> (109.2586, 384.0451) construction
  line L64 (109.2586, 384.0451) -> (97.648, 384.0451) construction
  line L65 (97.648, 384.0451) -> (97.648, 387.5837) construction
  line L66 (167.5218, 387.5837) -> (183.876, 387.5837) construction
  line L67 (183.876, 387.5837) -> (183.876, 362.5837) construction
  line L68 (183.876, 362.5837) -> (178.6733, 362.5837) construction
  line L69 (178.6733, 362.5837) -> (178.6733, 384.0451) construction
  line L70 (178.6733, 384.0451) -> (167.5218, 384.0451) construction
  line L71 (167.5218, 384.0451) -> (167.5218, 387.5837) construction
  line L72 (244.2796, 191.5951) -> (151.7796, 138.1902) construction
  line L73 (151.7796, 138.1902) -> (59.2796, 191.5951) construction
  line L74 (59.2796, 191.5951) -> (59.2796, 298.4049) construction
  line L75 (59.2796, 298.4049) -> (151.7796, 351.8098) construction
  line L76 (151.7796, 351.8098) -> (244.2796, 298.4049) construction
  line L77 (244.2796, 298.4049) -> (244.2796, 191.5951) construction
  line L78 (205.0313, 387.3542) -> (205.0313, 383.0696) construction
  line L79 (197.2272, 377.4077) -> (198.9104, 376.4705) construction
  line L80 (189.9204, 362.8324) -> (189.9204, 366.8301) construction
  line L81 (196.4047, 371.8989) -> (194.6067, 372.8936) construction
  line L82 (162.7207, 387.5837) -> (166.508, 387.5837) construction
  line L83 (166.508, 387.5837) -> (156.8102, 362.5837) construction
  line L84 (156.8102, 362.5837) -> (151.5883, 362.5837) construction
  line L85 (151.5883, 362.5837) -> (141.8523, 387.5837) construction
  line L86 (141.8523, 387.5837) -> (147.1889, 387.5837) construction
  line L87 (147.1889, 387.5837) -> (149.7903, 380.9081) construction
  line L88 (149.7903, 380.9081) -> (160.1193, 380.9081) construction
  line L89 (160.1193, 380.9081) -> (162.7207, 387.5837) construction
  line L90 (126.8944, 387.5837) -> (132.0971, 387.5837) construction
  line L91 (132.0971, 387.5837) -> (132.0971, 366.0267) construction
  line L92 (132.0971, 366.0267) -> (141.0489, 366.0267) construction
  line L93 (141.0489, 366.0267) -> (141.0489, 362.5837) construction
  line L94 (141.0489, 362.5837) -> (117.9426, 362.5837) construction
  line L95 (117.9426, 362.5837) -> (117.9426, 366.0267) construction
  line L96 (117.9426, 366.0267) -> (126.8944, 366.0267) construction
  line L97 (126.8944, 366.0267) -> (126.8944, 387.5837) construction
  line L98 (234.8993, 427.5402) -> (239.7961, 427.5402) construction
  line L99 (239.7961, 427.5402) -> (239.7961, 402.5402) construction
  line L100 (239.7961, 402.5402) -> (230.4426, 402.5402) construction
  line L101 (227.669, 415.8723) -> (219.5015, 427.5402) construction
  line L102 (219.5015, 427.5402) -> (225.8328, 427.5402) construction
  line L103 (225.8328, 427.5402) -> (232.0493, 417.326) construction
  line L104 (232.0493, 417.326) -> (234.8993, 417.326) construction
  line L105 (234.8993, 417.326) -> (234.8993, 427.5402) construction
  line L106 (178.262, 427.5402) -> (187.4816, 427.5402) construction
  line L107 (187.4816, 427.5402) -> (187.4816, 402.5402) construction
  line L108 (187.4816, 402.5402) -> (179.0462, 402.5402) construction
  line L109 (108.1778, 427.5402) -> (113.3806, 427.5402) construction
  line L110 (113.3806, 427.5402) -> (113.3806, 402.5402) construction
  line L111 (113.3806, 402.5402) -> (108.1778, 402.5402) construction
  line L112 (108.1778, 402.5402) -> (108.1778, 427.5402) construction
  line L113 (78.6828, 427.3107) -> (78.6828, 423.0261) construction
  line L114 (70.8787, 417.3642) -> (72.5619, 416.427) construction
  line L115 (63.5719, 402.7889) -> (63.5719, 406.7866) construction
  line L116 (70.0562, 411.8554) -> (68.2582, 412.8501) construction
  line L117 (156.1065, 467.5284) -> (159.645, 467.5284) construction
  line L118 (159.645, 467.5284) -> (154.6642, 442.5284) construction
  line L119 (154.6642, 442.5284) -> (147.1258, 442.5284) construction
  line L120 (147.3373, 455.5861) -> (141.395, 467.5284) construction
  line L121 (141.395, 467.5284) -> (145.3181, 467.5284) construction
  line L122 (145.3181, 467.5284) -> (150.5681, 456.4707) construction
  line L123 (150.5681, 456.4707) -> (153.9142, 456.4707) construction
  line L124 (153.9142, 456.4707) -> (156.1065, 467.5284) construction
  line L125 (122.8181, 467.5284) -> (137.7027, 467.5284) construction
  line L126 (137.7027, 467.5284) -> (137.1642, 464.8361) construction
  line L127 (130.4719, 457.6438) -> (128.3758, 456.0476) construction
  line L128 (133.0873, 446.4515) -> (132.4912, 443.4707) construction
  line L129 (125.645, 457.2207) -> (127.7412, 458.7399) construction
  line L130 (133.1835, 464.6245) -> (122.2219, 464.6245) construction
  line L131 (122.2219, 464.6245) -> (122.8181, 467.5284) construction
  line L132 (305.8043, 541.9951) -> (305.8043, -2.2451) construction
  line L133 (305.8043, -2.2451) -> (252.4045, -2.2451) construction
  line L134 (252.4045, -2.2451) -> (252.4045, 5.3749) construction
  line L135 (252.4045, 5.3749) -> (228.9547, 5.3749) construction
  line L136 (228.9547, 5.3749) -> (228.9547, -2.2451) construction
  line L137 (228.9547, -2.2451) -> (74.6045, -2.2451) construction
  line L138 (74.6045, -2.2451) -> (74.6045, 5.3749) construction
  line L139 (74.6045, 5.3749) -> (51.1547, 5.3749) construction
  line L140 (51.1547, 5.3749) -> (51.1547, -2.2451) construction
  line L141 (51.1547, -2.2451) -> (-2.2451, -2.2451) construction
  line L142 (-2.2451, -2.2451) -> (-2.2451, 541.9951) construction
  line L143 (-2.2451, 541.9951) -> (51.1547, 541.9951) construction
  line L144 (51.1547, 541.9951) -> (51.1547, 534.3751) construction
  line L145 (51.1547, 534.3751) -> (74.6045, 534.3751) construction
  line L146 (74.6045, 534.3751) -> (74.6045, 541.9951) construction
  line L147 (74.6045, 541.9951) -> (228.9547, 541.9951) construction
  line L148 (228.9547, 541.9951) -> (228.9547, 534.3751) construction
  line L149 (228.9547, 534.3751) -> (252.4045, 534.3751) construction
  line L150 (252.4045, 534.3751) -> (252.4045, 541.9951) construction
  line L151 (252.4045, 541.9951) -> (305.8043, 541.9951) construction
  line L152 (252.4045, 329.2249) -> (252.4045, 324.8251) construction
  line L153 (252.4045, 324.8251) -> (228.9547, 324.8251) construction
  line L154 (228.9547, 324.8251) -> (228.9547, 329.2249) construction
  line L155 (228.9547, 329.2249) -> (252.4045, 329.2249) construction
  line L156 (252.4045, 176.8249) -> (252.4045, 172.4251) construction
  line L157 (252.4045, 172.4251) -> (228.9547, 172.4251) construction
  line L158 (228.9547, 172.4251) -> (228.9547, 176.8249) construction
  line L159 (228.9547, 176.8249) -> (252.4045, 176.8249) construction
  line L160 (74.6045, 176.8249) -> (51.1547, 176.8249) construction
  line L161 (51.1547, 176.8249) -> (51.1547, 172.4251) construction
  line L162 (51.1547, 172.4251) -> (74.6045, 172.4251) construction
  line L163 (74.6045, 172.4251) -> (74.6045, 176.8249) construction
  line L164 (74.6045, 329.2249) -> (51.1547, 329.2249) construction
  line L165 (51.1547, 329.2249) -> (51.1547, 324.8251) construction
  line L166 (51.1547, 324.8251) -> (74.6045, 324.8251) construction
  line L167 (74.6045, 324.8251) -> (74.6045, 329.2249) construction
  line L168 (254.6496, 532.13) -> (226.7096, 532.13) projected
  circle A14 centre (228.9547, 534.3751) radius 3.175
  circle A15 centre (252.4045, 534.3751) radius 3.175
  circle A16 centre (74.6045, 534.3751) radius 3.175
  circle A17 centre (51.1547, 534.3751) radius 3.175
  line L169 (226.7096, 7.62) -> (226.7096, 0) projected
  circle A18 centre (228.9547, 5.3749) radius 3.175
  circle A19 centre (252.4045, 5.3749) radius 3.175
  circle A20 centre (51.1547, 5.3749) radius 3.175
  circle A21 centre (74.6045, 5.3749) radius 3.175
  line L170 (48.9096, 179.07) -> (76.8496, 179.07) projected
  circle A22 centre (51.1547, 176.8249) radius 3.175
  circle A23 centre (51.1547, 172.4251) radius 3.175
  circle A24 centre (74.6045, 172.4251) radius 3.175
  circle A25 centre (74.6045, 176.8249) radius 3.175
  circle A26 centre (51.1547, 329.2249) radius 3.175
  circle A27 centre (51.1547, 324.8251) radius 3.175
  line L171 (76.8496, 322.58) -> (48.9096, 322.58) projected
  circle A28 centre (74.6045, 324.8251) radius 3.175
  circle A29 centre (74.6045, 329.2249) radius 3.175
  circle A30 centre (228.9547, 329.2249) radius 3.175
  circle A31 centre (228.9547, 324.8251) radius 3.175
  circle A32 centre (252.4045, 329.2249) radius 3.175
  circle A33 centre (252.4045, 324.8251) radius 3.175
  circle A34 centre (228.9547, 176.8249) radius 3.175
  circle A35 centre (228.9547, 172.4251) radius 3.175
  circle A36 centre (252.4045, 172.4251) radius 3.175
  line L172 (254.6496, 179.07) -> (254.6496, 170.18) projected
  circle A37 centre (252.4045, 176.8249) radius 3.175
  dimension "d78" = 6.35
  dimension "d79" = 6.35
  dimension "d80" = 6.35
  dimension "d81" = 6.35
  dimension "d82" = 6.35
  constraints: 72 end point, 23 coincident, 171 other
extrude "Extrusion10" cut sketch "Sketch10" against normal through all
equation "\"d2\" = Panel_Thickness"
equation "\"d8\" = Panel_Thickness + Fit_Tolerance"
equation "\"d14\" = Panel_Thickness + Fit_Tolerance"
equation "\"d16\" = Panel_Thickness"
equation "\"d18\" = Panel_Thickness"
equation "\"d23\" = Panel_Thickness"
equation "\"d25\" = Panel_Thickness"
equation "\"d68\" = Fit_Tolerance"
equation "\"d69\" = Fit_Tolerance"
equation "\"d70\" = Fit_Tolerance"
equation "\"d71\" = Fit_Tolerance"
equation "\"d72\" = Fit_Tolerance"
equation "\"d73\" = Fit_Tolerance"
equation "\"d74\" = Fit_Tolerance"
equation "\"d75\" = Fit_Tolerance"
equation "\"d78\" = Tool_Dia"
equation "\"d79\" = Tool_Dia"
equation "\"d80\" = Tool_Dia"
equation "\"d81\" = Tool_Dia"
equation "\"d82\" = Tool_Dia"
equation "\"Panel_Thickness\" = 6.35"
equation "\"Fit_Tolerance\" = 1.27"
equation "\"Tool_Dia\" = 6.35"
body "Solid1"
